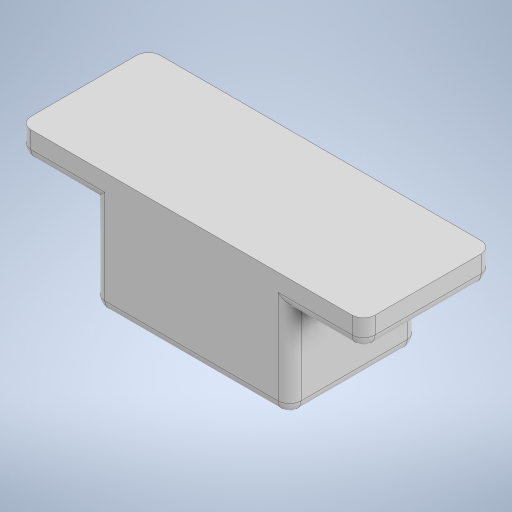
# Autodesk Inventor part: Platform
Saved by Autodesk Inventor 2024 (Build 280153000, 153)
## iProperties
Created: 2024-04-30
Part Number: Platform
Material: Generic
Document SubType Name: Modeling
Designer: cyan924
Density: 1 g/cm^3
Appearance: Default
Author: cyan924
Autodesk Inventor part; units mm, degrees
ref_plane "YZ Plane" through (0, 0, 0) normal (1, 0, 0) x (0, 1, 0)
ref_plane "XZ Plane" through (0, 0, 0) normal (0, 1, 0) x (-1, 0, 0)
ref_plane "XY Plane" through (0, 0, 0) normal (0, 0, 1) x (1, 0, 0)
sketch "Sketch1" plane through (0, 0, 0) normal (0, 1, 0) x (-1, 0, 0)
  line L0 (0, 0) -> (34.2, 0)
  line L1 (34.2, 0) -> (34.2, -22.5)
  line L2 (34.2, -22.5) -> (0, -22.5)
  line L3 (0, -22.5) -> (0, 0)
  line L4 (5, -17.5) -> (29.2, -17.5)
  line L5 (29.2, -17.5) -> (29.2, -5)
  line L6 (29.2, -5) -> (5, -5)
  line L7 (5, -5) -> (5, -17.5)
  dimension "d64" = 24.2
  dimension "d65" = 12.5
  dimension "d66" = 5
  dimension "d67" = 5
  dimension "d68" = 5
  dimension "d69" = 5
  constraints: 16 end point, 4 parallel, 2 horizontal, 2 perpendicular
  measures "d64" distance between parallel lines of L5 L7
  measures "d65" distance of L4.end L5.end
  measures "d66" distance between parallel lines of L1 L5
  measures "d67" distance between parallel lines of L3 L7
  measures "d68" distance between parallel lines of L0 L6
  measures "d69" distance between parallel lines of L2 L4
extrude "Extrusion4" add sketch "Sketch1" along normal blind 16.4
sketch "Sketch6" plane through (0, 16.4, 0) normal (0, 1, 0) x (1, 0, 0)
  line L0 (0, 0) -> (0, 22.5) projected
  line L1 (-34.2, 0) -> (0, 0) projected
  line L2 (-47.1, 22.5) -> (12.9, 22.5)
  line L3 (12.9, 22.5) -> (12.9, 0)
  line L4 (12.9, 0) -> (-47.1, 0)
  line L5 (-47.1, 0) -> (-47.1, 22.5)
  line L6 (0, 22.5) -> (-34.2, 22.5) projected
  point P0 (-17.1, 0)
  point P1 (15.9799, 21.8)
  point P2 (-17.1, 22.5)
  point P3 (-17.1, 22.5)
  dimension "d75" = 60
  dimension "d77" = 0
  constraints: 8 end point, 2 midpoint, 2 parallel, 1 horizontal, 1 perpendicular, 2 other
  measures "d75" distance between parallel lines of L3 L5
  measures "d77" distance of point (-17.1, 22.5) point (-17.1, 22.5)
extrude "Extrusion6" add sketch "Sketch6" along normal blind 5
sketch "Sketch8" plane through (-34.2, 0, -22.5) normal (-1, 0, 0) x (0, 0, 1)
  line L0 (17.5, 0) -> (17.5, 16.4) projected
  line L1 (5, 16.4) -> (17.5, 16.4) projected
  line L2 (17.5, 6.4) -> (5, 6.4)
  line L3 (5, 6.4) -> (5, 16.4)
  line L4 (5, 16.4) -> (17.5, 16.4)
  line L5 (17.5, 16.4) -> (17.5, 6.4)
  point P0 (22.5, 0)
  dimension "d176" = 10
  constraints: 8 end point, 2 parallel, 1 horizontal, 1 perpendicular, 1 point on line
  measures "d176" distance between parallel lines of L1 L2
extrude "Extrusion8" cut sketch "Sketch8" against normal blind 7.5
fillet "Fillet2" radius 2 21 edges at (-17.1, 0, -22.5) (-34.2, 0, -11.25) (0, 0, -11.25) (-17.1, 0, 0) (0, 8.2, -22.5) (6.45, 16.4, -22.5) (12.9, 16.4, -11.25) (6.45, 16.4, 0) (0, 8.2, 0) (-34.2, 8.2, -22.5) (-40.65, 16.4, -22.5) (-47.1, 16.4, -11.25) (-40.65, 16.4, 0) (-34.2, 8.2, 0) (12.9, 18.9, -22.5) (12.9, 18.9, 0) (-47.1, 18.9, -22.5) (-47.1, 18.9, 0) (-34.2, 11.4, -5) (-34.2, 6.4, -11.25) (-34.2, 11.4, -17.5)
equation "\"box\" = 4.5"
equation "\"walllength\" = 1"
equation "\"gap\" = 8.1"
equation "\"d34\" = 4.6"
equation "\"d35\" = 8"
equation "\"offset\" = 5"
equation "\"d44\" = 4.6"
equation "\"d89\" = 4.6"
equation "\"d126\" = 4.6"
equation "\"d134\" = 4.6"
equation "\"d135\" = 8"
equation "\"d140\" = 4.6"
equation "\"d144\" = 4.6"
equation "\"d162\" = 4.6"
equation "\"d163\" = 4.6"
equation "\"d164\" = 8"
equation "\"d165\" = 4.6"
equation "\"d166\" = 4.6"
equation "\"d167\" = 4.6"
body "Solid2"
